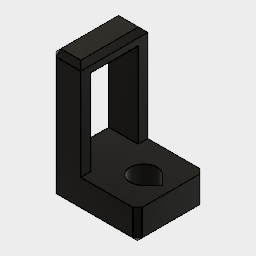
Pelvis (x4) (Autodesk Fusion 360 design; units mm, degrees)
Autodesk Fusion 360 part; units mm, degrees
sketch "Sketch1" plane through (0, 0, 0) normal (0, 1, 0) x (1, 0, 0)
  line L0 (0, 0) -> (23, 0)
  line L1 (23, 0) -> (23, 13)
  line L2 (23, 13) -> (0, 13)
  line L3 (0, 13) -> (0, 0)
  line L4 (23, 6.5) -> (15.5, 6.5)
  circle A0 centre (15.5, 6.5) radius 3.5
  line L5 (15.5, 6.5) -> (15.5, 10)
  line L6 (15.5, 6.5) -> (15.5, 3)
  line L7 (15.5, 6.5) -> (15.4844, 11.45)
  line L8 (15.4844, 11.45) -> (20.4344, 6.5)
  line L9 (15.4844, 11.45) -> (22.2175, 11.45) construction
  line L10 (15.5, 1.5) -> (22.8389, 1.5) construction
  line L11 (15.5, 6.5) -> (15.4844, 1.55)
  line L12 (15.4844, 1.55) -> (20.4344, 6.5)
  dimension "d1" = 23
  dimension "d2" = 13
  dimension "d16" = 7.5
  dimension "d17" = 7
  dimension "d18" = 4.95
  dimension "d19" = 45
  measures "d1" distance of L0.start L0.end
  measures "d2" distance of L0.start L2.end
  measures "d16" distance of L4.start L4.end
  measures "d17" diameter of A0
  measures "d18" distance of L4.end L7.end
  measures "d19" angle of L8 L9
sketch "Sketch2" plane through (0, 0, 0) normal (0, 1, 0) x (1, 0, 0)
  line L0 (0, 0) -> (0, -2.5)
  line L1 (0, 13) -> (0, 15.5)
  line L2 (0, -2.5) -> (23, -2.5)
  line L3 (23, -2.5) -> (23, 15.5)
  line L4 (23, 15.5) -> (0, 15.5)
  line L5 (0, 15.5) -> (0, -2.5)
  point P0 (0, 13)
  dimension "d3" = 2.5
  dimension "d4" = 2.5
  dimension "d5" = 23
  measures "d3" distance of L0.start L0.end
  measures "d4" distance of P0 L1.end
  measures "d5" distance of L0.end L2.end
extrude "Extrude1" add sketch "Sketch2" against normal blind 4
sketch "Sketch3" plane through (0, 0, 0) normal (0, 1, 0) x (-1, 0, 0)
  line L0 (0, -15.5) -> (0, 2.5)
  line L1 (0, 2.5) -> (-23, 2.5)
  line L2 (-23, 2.5) -> (-23, -15.5)
  line L3 (-23, -15.5) -> (0, -15.5)
  line L4 (0, 2.5) -> (-7, 2.5)
  line L5 (-7, 2.5) -> (-7, 0)
  line L6 (-7, 0) -> (0, 0)
  line L7 (0, 0) -> (0, 2.5)
  line L8 (0, -13) -> (-7, -13)
  line L9 (-7, -13) -> (-7, -15.5)
  line L10 (-7, -15.5) -> (0, -15.5)
  line L11 (0, -15.5) -> (0, -13)
  point P0 (0, -13)
  dimension "d8" = 7
  dimension "d9" = 7
  measures "d8" distance of L0.end L4.end
  measures "d9" distance of P0 L8.end
extrude "Extrude2" add sketch "Sketch3" along normal blind 15.75 contours L0 L3 L8 L9 L10 L11 | L0 L1 L4 L5 L6 L7
extrude "Extrude3" add 2 faces at (2.3333, 15.75, 0.8333) (2.3333, 15.75, -14.6667) along direction (0, 1, 0) blind 6.75
sketch "Sketch4" plane through (0, 22.5, 0) normal (0, 1, 0) x (-1, 0, 0)
  line L0 (0, 0) -> (0, 2.5)
  line L1 (0, 2.5) -> (-7, 2.5)
  line L2 (-7, 2.5) -> (-7, 0)
  line L3 (-7, 0) -> (0, 0)
  line L4 (0, 2.5) -> (-7, 2.5)
  line L5 (-7, 2.5) -> (-7, -15.5)
  line L6 (-7, -15.5) -> (0, -15.5)
  line L7 (0, -15.5) -> (0, 2.5)
  point P0 (-7, -15.5)
extrude "Extrude4" add sketch "Sketch4" along normal blind 3
extrude "Extrude5" cut sketch "Sketch1" against normal blind 6 contours L4 A0 L12 | L4 A0 L8 | L4 A0 L6 L12 | L4 A0 L5 L8 | A0 L7 L11
delete_face "DeleteFace1" 1 faces at (15.5, -1.3333, -7.6667)
delete_face "DeleteFace2" 1 faces at (15.5, -1.3333, -5.3333)
extrude "Extrude6" add 1 faces at (7, 24.5, -8.6667) along direction (1, 0, 0) blind 0.5
extrude "Extrude7" add 1 faces at (7.5, 24.5, -8.6667) along direction (1, 0, 0) blind 0.3
extrude "Extrude8" add 1 faces at (2.6, 7.5, -13) along direction (0, 0, 1) blind 0.5
extrude "Extrude9" add 1 faces at (2.6, 15, 0) along direction (0, 0, -1) blind 0.5
extrude "Extrude10" cut 1 faces at (2.6, 15, -0.5) along direction (0, 0, 1) blind 0.25
extrude "Extrude11" cut 1 faces at (2.6, 7.5, -12.5) along direction (0, 0, -1) blind 0.25
sketch "Sketch5" plane through (7.8, 0, 0) normal (1, 0, 0) x (0, 0, -1)
  line L0 (12.75, 22.5) -> (12.75, 0)
  line L1 (12.75, 0) -> (15.5, 0)
  line L2 (15.5, 0) -> (15.5, 25.5)
  line L3 (15.5, 25.5) -> (-2.5, 25.5)
  line L4 (-2.5, 25.5) -> (-2.5, 0)
  line L5 (-2.5, 0) -> (0.25, 0)
  line L6 (0.25, 0) -> (0.25, 22.5)
  line L7 (0.25, 22.5) -> (12.75, 22.5)
  line L8 (-2.5, 25.5) -> (-2.5, 22.5)
  line L9 (-2.5, 22.5) -> (15.5012, 22.5)
  dimension "d36" = 3
  measures "d36" distance of L3.end L8.end
extrude "Extrude13" cut 1 faces at (2.6, 7.1667, 2.5) along direction (0, 0, -1) blind 0.125
extrude "Extrude14" cut 1 faces at (2.6, 7.1667, -15.5) along direction (0, 0, 1) blind 0.125
extrude "Extrude15" cut 1 faces at (23, -2.6667, -3.5417) along direction (-1, 0, 0) blind 0.25
sketch "Sketch6" plane through (0, 0, 0) normal (0, 1, 0) x (-1, 0, 0)
  line L0 (-22.75, 2.375) -> (-22.75, -15.375)
  line L1 (-22.75, -15.375) -> (-7.8, -15.375)
  line L2 (-7.8, -15.375) -> (-7.8, -12.75)
  line L3 (-7.8, -12.75) -> (0, -12.75)
  line L4 (0, -12.75) -> (0, -0.25)
  line L5 (0, -0.25) -> (-7.8, -0.25)
  line L6 (-7.8, -0.25) -> (-7.8, 2.375)
  line L7 (-7.8, 2.375) -> (-22.75, 2.375)
  arc A0 (-17.7726, -9.1618) -> (-17.7726, -3.8382) centre (-15.5, -6.5) ccw
  line L8 (-17.7726, -9.1618) -> (-20.4344, -6.5)
  line L9 (-20.4344, -6.5) -> (-17.7726, -3.8382)
  line L10 (-15.5, -6.5) -> (-22.75, -6.5)
extrude "Extrude16" add 1 faces at (4.0031, -4, -6.4144) along direction (0, -1, 0) blind 4.25
chamfer "Chamfer2" distance 1.25 angle 45 12 edges at (0, 8.625, -15.375) (3.9, 25.5, -15.375) (0, 25.5, -6.5) (3.9, 25.5, 2.375) (0, 8.625, 2.375) (7.8, 25.5, -6.5) (11.375, -8.25, 2.375) (22.75, -4.125, 2.375) (22.75, -4.125, -15.375) (11.375, -8.25, -15.375) (22.75, -8.25, -6.5) (0, -8.25, -6.5)
chamfer "Chamfer1" [suppressed]
